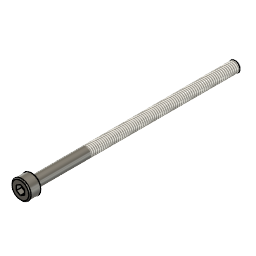
Equatorial Mount (Autodesk Fusion 360 archive; units mm, degrees)
design "Hexagon Socket Head Cap Screw ISO 4762 - M4 x 75 Steel 4.6 Plain"
description: Hexagon Socket Head Cap Screw ISO 4762 - M4 x 75
part number: ISO 4762 - M4 x 75 Steel 4.6 Plain
Autodesk Fusion 360 part; units mm, degrees
note: some values were not read from the file. Chosen so that the rebuilt part matches the saved one: how an offset face is resized. Set by a fixed rule: which face or edge a step refers to; which sketch regions a step uses.
sketch "Sketch1" plane through (0, 0, 0) normal (0, 1, 0) x (1, 0, 0)
  line L0 (-2, 0) -> (-2, 75)
  line L1 (-2, 75) -> (0, 75)
  line L2 (0, 75) -> (0, -4)
  line L3 (-2, 0) -> (-3.5, 0)
  line L4 (-3.5, 0) -> (-3.5, -4)
  line L5 (-3.5, -4) -> (0, -4)
  dimension "d9" = 4
  dimension "d106" = 4
  dimension "d107" = 75
  dimension "d116" = 7
  constraint perpendicular L0 L1
  constraint collinear origin L1.end L2.end
  constraint perpendicular L0 L3
  constraint coincident origin L3
  constraint vertical L2
  constraint coincident L2 L5.end
  constraint perpendicular L2 L5
  measures "d106" distance of L3 L5
  measures "d107" distance of origin L1
revolve "Revolve1" add sketch "Sketch1" angle 360 about axis through (0, 0, -75) along (0, 0, 1)
ref_plane "WorkPlane1" through (0, 0, 4) normal (0, 0, 1) x (1, 0, 0)
sketch "Sketch6" plane through (0, 0, 4) normal (0, 0, 1) x (1, 0, 0)
  line L0 (-1.5, 0.866) -> (-1.5, -0.866)
  line L1 (-1.5, -0.866) -> (0, -1.7321)
  line L2 (0, -1.7321) -> (1.5, -0.866)
  line L3 (1.5, -0.866) -> (1.5, 0.866)
  line L4 (1.5, 0.866) -> (0, 1.7321)
  line L5 (0, 1.7321) -> (-1.5, 0.866)
  dimension "d117" = 3
  constraint vertical L0
  measures "d117" distance of L0 L3
extrude "Extrude1" cut sketch "Sketch6" against normal blind 2
extrude "Extrude2" cut 1 faces at (0, -0.5774, 2) along direction (0, 0, -1) blind 2 draft -85
fillet "Fillet4" radius 0.4 1 edges at (-3.2631, 1.2657, 4)
thread "Thread3" "ISO Metric profile 4.0 M4x0.7 M4x0.7 6g" major diameter 3.908 minor diameter 3.111 pitch 0.7 angle 60 resizes the face on face at (-1.9901, 0.1991, -50)
sketch "Sketch7" plane through (0, 0, 0) normal (0, 1, 0) x (1, 0, 0)
  line L0 (-2.04, 75) -> (-2.04, 74.6)
  line L1 (-2.04, 74.6) -> (-1.64, 75)
  line L2 (0, 75) -> (0, -4)
  line L3 (-2.04, 75) -> (0, 75)
  dimension "d101" = 45
  dimension "d112" = 0.4
  dimension "d113" = 2.04
  constraint coincident L2.start L3.end
  constraint perpendicular L2 L3
  constraint coincident L1.end L3
  constraint perpendicular L0 L3
  measures "d101" angle of L0 L1
  measures "d112" distance of L0.end L3
  measures "d113" distance of L0 L2.start
revolve "Revolve3" cut sketch "Sketch7" angle 360 about axis through (0, 0, 1.75) along (0, 0, 1)
equation "d9 = adsk_nomdia"
equation "adsk_nomlen = 75.00 mm"
equation "adsk_headh = 4.00 mm"
equation "adsk_headdia = 7.00 mm"
equation "adsk_nomdia = 4.00 mm"
equation "adsk_philwidth = 3.00 mm"
equation "d31 = -adsk_phildepth"
equation "adsk_phildepth = 2.00 mm"
equation "d71 = adsk_headh"
equation "d76 = -adsk_phildepth"
equation "adsk_thrlen = 55.00 mm"
equation "d86 = adsk_nomdia * 0.1"
equation "adsk_startang = 45.00 deg"
equation "d101 = adsk_startang"
equation "adsk_pitch1 = 0.70 mm"
equation "adsk_startlen = 0.40 mm"
equation "d106 = adsk_headh"
equation "d107 = adsk_nomlen"
equation "d112 = adsk_startlen"
equation "d113 = adsk_nomdia * 0.51"
equation "d115 = min(adsk_thrlen; adsk_nomlen - 0.001 mm)"
equation "d116 = adsk_headdia"
equation "d117 = adsk_philwidth"

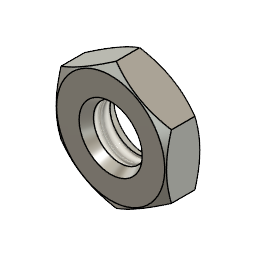
design "Hexagon Thin Nut ISO 4035 - M4 Steel 6 Plain"
description: Hexagon Thin Nut ISO 4035 - M4
part number: ISO 4035 - M4 Steel 6 Plain
Autodesk Fusion 360 part; units mm, degrees
sketch "Sketch1" plane through (0, 0, 0) normal (0, 1, 0) x (1, 0, 0)
  line L0 (0, 0) -> (0, -2.2)
  line L1 (-2, 0) -> (-3.43, 0)
  line L2 (-3.43, 0) -> (-4.0425, -0.3536)
  line L3 (-4.0425, -0.3536) -> (-4.0425, -1.8464)
  line L4 (-4.0425, -1.8464) -> (-3.43, -2.2)
  line L5 (-3.43, -2.2) -> (-2, -2.2)
  line L6 (-2, -2.2) -> (-2, 0)
  dimension "d121" = 4
  dimension "d122" = 30
  dimension "d123" = 30
  dimension "d128" = 8.085
  dimension "d172" = 6.86
  dimension "d179" = 2.2
  constraint vertical L0
  constraint coincident L0 L0.end
  constraint coincident origin L0
  constraint horizontal L1
  constraint coincident L0.start L1
  constraint coincident L0.start origin
  constraint coincident L0.end L5
  constraint vertical L1.end L4.end
  measures "d122" angle of L1 L2
  measures "d123" angle of L4 L5
  measures "d179" distance of L1 L5
revolve "Revolve1" add sketch "Sketch1" angle 360 about axis through (0, 0, 0) along (0, 0, 1)
sketch "Sketch8" plane through (0, 0, 2.2) normal (0, 0, 1) x (1, 0, 0)
  line L0 (-3.5, -2.0228) -> (-3.5, 2.0228)
  circle A0 centre (0, 0) radius 2
  circle A1 centre (0, 0) radius 4.0425
  dimension "d114" = 3.5
  constraint coincident L0.end A1
  constraint coincident L0.start A1
  constraint vertical L0
  measures "d114" distance of A0.centre L0
extrude "Extrude5" cut sketch "Sketch8" against normal blind 2.2 contours L0 A1 picked at (-3.5875, 0.4927)
pattern_circular "C-Pattern2" count 6 over 360 about axis through (0, 0, 1.75) along (0, 0, 1) of "Extrude5"
thread "Thread3" "ISO Metric profile 4.0 M4x0.7 M4x0.7 6H" major diameter 4.1095 minor diameter 3.332 pitch 0.7 angle 60 resizes the face on face at (-1.9975, 0.0997, 1.4667)
sketch "Sketch12" plane through (0, 0, 0) normal (0, 1, 0) x (1, 0, 0)
  line L0 (-2, 0) -> (0, 0)
  line L1 (-1.3649, -1.1) -> (-2, 0)
  line L2 (-2, -2.2) -> (0, -2.2)
  line L3 (-1.3649, -1.1) -> (-2, -2.2)
  line L4 (0, 0) -> (0, -2.2)
  dimension "d169" = 60
  dimension "d177" = 2
  dimension "d178" = 60
  constraint horizontal L0
  constraint coincident L1.start L3.start
  constraint vertical L0.start L2.start
  constraint coincident L2.end L4.end
  constraint coincident L0.end L4.start
  constraint perpendicular L2 L4
  measures "d169" angle of L2 L3
  measures "d177" distance of L0.start L4
  measures "d178" angle of L0 L1
revolve "Revolve3" cut sketch "Sketch12" angle 360 about axis through (0, 0, 1.75) along (0, 0, 1)
equation "adsk_nheig = 2.20 mm"
equation "adsk_maxdia = 8.085 mm"
equation "adsk_nomdia = 4.00 mm"
equation "d89 = -adsk_nheig"
equation "adsk_waflat = 7.00 mm"
equation "d114 = adsk_waflat / 2"
equation "adsk_chamang1 = 30.00 deg"
equation "adsk_chamang2 = 30.00 deg"
equation "d121 = adsk_nomdia"
equation "d122 = adsk_chamang1"
equation "d123 = adsk_chamang2"
equation "d128 = adsk_maxdia"
equation "d163 = adsk_nheig"
equation "adsk_beardia = 6.86 mm"
equation "d172 = adsk_beardia"
equation "d177 = adsk_nomdia * 0.5"
equation "d179 = adsk_nheig"

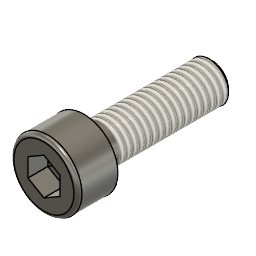
design "Hexagon Socket Head Cap Screw ISO 4762 - M5 x 16 Steel 4.6 Plain"
description: Hexagon Socket Head Cap Screw ISO 4762 - M5 x 16
part number: ISO 4762 - M5 x 16 Steel 4.6 Plain
Autodesk Fusion 360 part; units mm, degrees
sketch "Sketch1" plane through (0, 0, 0) normal (0, 1, 0) x (1, 0, 0)
  line L0 (-2.5, 0) -> (-2.5, 16)
  line L1 (-2.5, 16) -> (0, 16)
  line L2 (0, 16) -> (0, -5)
  line L3 (-2.5, 0) -> (-4.25, 0)
  line L4 (-4.25, 0) -> (-4.25, -5)
  line L5 (-4.25, -5) -> (0, -5)
  dimension "d9" = 5
  dimension "d106" = 5
  dimension "d107" = 16
  dimension "d116" = 8.5
  constraint perpendicular L0 L1
  constraint collinear origin L1.end L2.end
  constraint perpendicular L0 L3
  constraint coincident origin L3
  constraint vertical L2
  constraint coincident L2 L5.end
  constraint perpendicular L2 L5
  measures "d106" distance of L3 L5
  measures "d107" distance of origin L1
revolve "Revolve1" add sketch "Sketch1" angle 360 about axis through (0, 0, -16) along (0, 0, 1)
ref_plane "WorkPlane1" through (0, 0, 5) normal (0, 0, 1) x (1, 0, 0)
sketch "Sketch6" plane through (0, 0, 5) normal (0, 0, 1) x (1, 0, 0)
  line L0 (-2, 1.1547) -> (-2, -1.1547)
  line L1 (-2, -1.1547) -> (0, -2.3094)
  line L2 (0, -2.3094) -> (2, -1.1547)
  line L3 (2, -1.1547) -> (2, 1.1547)
  line L4 (2, 1.1547) -> (0, 2.3094)
  line L5 (0, 2.3094) -> (-2, 1.1547)
  dimension "d117" = 4
  constraint vertical L0
  measures "d117" distance of L0 L3
extrude "Extrude1" cut sketch "Sketch6" against normal blind 2.5
extrude "Extrude2" cut 1 faces at (0.6667, -0.3849, 2.5) along direction (0, 0, -1) blind 2.5 draft -85
fillet "Fillet4" radius 0.5 1 edges at (-3.9624, 1.5369, 5)
thread "Thread3" "ISO Metric profile 5.0 M5x0.8 M5x0.8 6g" major diameter 4.901 minor diameter 3.9895 pitch 0.8 angle 60 resizes the face on face at (-2.4876, 0.2489, -10.6667)
sketch "Sketch7" plane through (0, 0, 0) normal (0, 1, 0) x (1, 0, 0)
  line L0 (-2.55, 16) -> (-2.55, 15.5)
  line L1 (-2.55, 15.5) -> (-2.05, 16)
  line L2 (0, 16) -> (0, -5)
  line L3 (-2.55, 16) -> (0, 16)
  dimension "d101" = 45
  dimension "d112" = 0.5
  dimension "d113" = 2.55
  constraint coincident L2.start L3.end
  constraint perpendicular L2 L3
  constraint coincident L1.end L3
  constraint perpendicular L0 L3
  measures "d101" angle of L0 L1
  measures "d112" distance of L0.end L3
  measures "d113" distance of L0 L2.start
revolve "Revolve3" cut sketch "Sketch7" angle 360 about axis through (0, 0, 1.75) along (0, 0, 1)
equation "d9 = adsk_nomdia"
equation "adsk_nomlen = 16.00 mm"
equation "adsk_headh = 5.00 mm"
equation "adsk_headdia = 8.50 mm"
equation "adsk_nomdia = 5.00 mm"
equation "adsk_philwidth = 4.00 mm"
equation "d31 = -adsk_phildepth"
equation "adsk_phildepth = 2.50 mm"
equation "d71 = adsk_headh"
equation "d76 = -adsk_phildepth"
equation "adsk_thrlen = 14.00 mm"
equation "d86 = adsk_nomdia * 0.1"
equation "adsk_startang = 45.00 deg"
equation "d101 = adsk_startang"
equation "adsk_pitch1 = 0.80 mm"
equation "adsk_startlen = 0.50 mm"
equation "d106 = adsk_headh"
equation "d107 = adsk_nomlen"
equation "d112 = adsk_startlen"
equation "d113 = adsk_nomdia * 0.51"
equation "d115 = min(adsk_thrlen; adsk_nomlen - 0.001 mm)"
equation "d116 = adsk_headdia"
equation "d117 = adsk_philwidth"

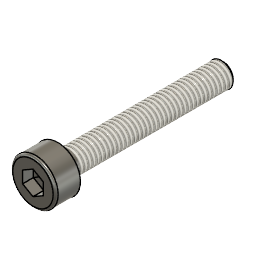
design "Hexagon Socket Head Cap Screw ISO 4762 - M3 x 20 Steel 4.6 Plain"
description: Hexagon Socket Head Cap Screw ISO 4762 - M3 x 20
part number: ISO 4762 - M3 x 20 Steel 4.6 Plain
Autodesk Fusion 360 part; units mm, degrees
sketch "Sketch1" plane through (0, 0, 0) normal (0, 1, 0) x (1, 0, 0)
  line L0 (-1.5, 0) -> (-1.5, 20)
  line L1 (-1.5, 20) -> (0, 20)
  line L2 (0, 20) -> (0, -3)
  line L3 (-1.5, 0) -> (-2.75, 0)
  line L4 (-2.75, 0) -> (-2.75, -3)
  line L5 (-2.75, -3) -> (0, -3)
  dimension "d9" = 3
  dimension "d106" = 3
  dimension "d107" = 20
  dimension "d116" = 5.5
  constraint perpendicular L0 L1
  constraint collinear origin L1.end L2.end
  constraint perpendicular L0 L3
  constraint coincident origin L3
  constraint vertical L2
  constraint coincident L2 L5.end
  constraint perpendicular L2 L5
  measures "d106" distance of L3 L5
  measures "d107" distance of origin L1
revolve "Revolve1" add sketch "Sketch1" angle 360 about axis through (0, 0, -20) along (0, 0, 1)
ref_plane "WorkPlane1" through (0, 0, 3) normal (0, 0, 1) x (1, 0, 0)
sketch "Sketch6" plane through (0, 0, 3) normal (0, 0, 1) x (1, 0, 0)
  line L0 (-1.25, 0.7217) -> (-1.25, -0.7217)
  line L1 (-1.25, -0.7217) -> (0, -1.4434)
  line L2 (0, -1.4434) -> (1.25, -0.7217)
  line L3 (1.25, -0.7217) -> (1.25, 0.7217)
  line L4 (1.25, 0.7217) -> (0, 1.4434)
  line L5 (0, 1.4434) -> (-1.25, 0.7217)
  dimension "d117" = 2.5
  constraint vertical L0
  measures "d117" distance of L0 L3
extrude "Extrude1" cut sketch "Sketch6" against normal blind 1.3
extrude "Extrude2" cut 1 faces at (-0.4167, 0.2406, 1.7) along direction (0, 0, -1) blind 1.3 draft -85
fillet "Fillet4" radius 0.3 1 edges at (-2.5639, 0.9944, 3)
thread "Thread3" "ISO Metric profile 3.0 M3x0.5 M3x0.5 6g" major diameter 2.927 minor diameter 2.3555 pitch 0.5 angle 60 resizes the face on face at (-1.4925, 0.1494, -13.3333)
sketch "Sketch7" plane through (0, 0, 0) normal (0, 1, 0) x (1, 0, 0)
  line L0 (-1.53, 20) -> (-1.53, 19.7)
  line L1 (-1.53, 19.7) -> (-1.23, 20)
  line L2 (0, 20) -> (0, -3)
  line L3 (-1.53, 20) -> (0, 20)
  dimension "d101" = 45
  dimension "d112" = 0.3
  dimension "d113" = 1.53
  constraint coincident L2.start L3.end
  constraint perpendicular L2 L3
  constraint coincident L1.end L3
  constraint perpendicular L0 L3
  measures "d101" angle of L0 L1
  measures "d112" distance of L0.end L3
  measures "d113" distance of L0 L2.start
revolve "Revolve3" cut sketch "Sketch7" angle 360 about axis through (0, 0, 1.75) along (0, 0, 1)
equation "d9 = adsk_nomdia"
equation "adsk_nomlen = 20.00 mm"
equation "adsk_headh = 3.00 mm"
equation "adsk_headdia = 5.50 mm"
equation "adsk_nomdia = 3.00 mm"
equation "adsk_philwidth = 2.50 mm"
equation "d31 = -adsk_phildepth"
equation "adsk_phildepth = 1.30 mm"
equation "d71 = adsk_headh"
equation "d76 = -adsk_phildepth"
equation "adsk_thrlen = 18.75 mm"
equation "d86 = adsk_nomdia * 0.1"
equation "adsk_startang = 45.00 deg"
equation "d101 = adsk_startang"
equation "adsk_pitch1 = 0.50 mm"
equation "adsk_startlen = 0.30 mm"
equation "d106 = adsk_headh"
equation "d107 = adsk_nomlen"
equation "d112 = adsk_startlen"
equation "d113 = adsk_nomdia * 0.51"
equation "d115 = min(adsk_thrlen; adsk_nomlen - 0.001 mm)"
equation "d116 = adsk_headdia"
equation "d117 = adsk_philwidth"

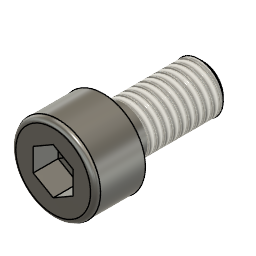
design "Hexagon Socket Head Cap Screw ISO 4762 - M5 x 10 Steel 4.6 Plain"
description: Hexagon Socket Head Cap Screw ISO 4762 - M5 x 10
part number: ISO 4762 - M5 x 10 Steel 4.6 Plain
Autodesk Fusion 360 part; units mm, degrees
sketch "Sketch1" plane through (0, 0, 0) normal (0, 1, 0) x (1, 0, 0)
  line L0 (-2.5, 0) -> (-2.5, 10)
  line L1 (-2.5, 10) -> (0, 10)
  line L2 (0, 10) -> (0, -5)
  line L3 (-2.5, 0) -> (-4.25, 0)
  line L4 (-4.25, 0) -> (-4.25, -5)
  line L5 (-4.25, -5) -> (0, -5)
  dimension "d9" = 5
  dimension "d106" = 5
  dimension "d107" = 10
  dimension "d116" = 8.5
  constraint perpendicular L0 L1
  constraint collinear origin L1.end L2.end
  constraint perpendicular L0 L3
  constraint coincident origin L3
  constraint vertical L2
  constraint coincident L2 L5.end
  constraint perpendicular L2 L5
  measures "d106" distance of L3 L5
  measures "d107" distance of origin L1
revolve "Revolve1" add sketch "Sketch1" angle 360 about axis through (0, 0, -10) along (0, 0, 1)
ref_plane "WorkPlane1" through (0, 0, 5) normal (0, 0, 1) x (1, 0, 0)
sketch "Sketch6" plane through (0, 0, 5) normal (0, 0, 1) x (1, 0, 0)
  line L0 (-2, 1.1547) -> (-2, -1.1547)
  line L1 (-2, -1.1547) -> (0, -2.3094)
  line L2 (0, -2.3094) -> (2, -1.1547)
  line L3 (2, -1.1547) -> (2, 1.1547)
  line L4 (2, 1.1547) -> (0, 2.3094)
  line L5 (0, 2.3094) -> (-2, 1.1547)
  dimension "d117" = 4
  constraint vertical L0
  measures "d117" distance of L0 L3
extrude "Extrude1" cut sketch "Sketch6" against normal blind 2.5
extrude "Extrude2" cut 1 faces at (0.6667, -0.3849, 2.5) along direction (0, 0, -1) blind 2.5 draft -85
fillet "Fillet4" radius 0.5 1 edges at (-3.9624, 1.5369, 5)
thread "Thread3" "ISO Metric profile 5.0 M5x0.8 M5x0.8 6g" major diameter 4.901 minor diameter 3.9895 pitch 0.8 angle 60 resizes the face on face at (-2.4876, 0.2489, -3.3333)
sketch "Sketch7" plane through (0, 0, 0) normal (0, 1, 0) x (1, 0, 0)
  line L0 (-2.55, 10) -> (-2.55, 9.5)
  line L1 (-2.55, 9.5) -> (-2.05, 10)
  line L2 (0, 10) -> (0, -5)
  line L3 (-2.55, 10) -> (0, 10)
  dimension "d101" = 45
  dimension "d112" = 0.5
  dimension "d113" = 2.55
  constraint coincident L2.start L3.end
  constraint perpendicular L2 L3
  constraint coincident L1.end L3
  constraint perpendicular L0 L3
  measures "d101" angle of L0 L1
  measures "d112" distance of L0.end L3
  measures "d113" distance of L0 L2.start
revolve "Revolve3" cut sketch "Sketch7" angle 360 about axis through (0, 0, 1.75) along (0, 0, 1)
equation "d9 = adsk_nomdia"
equation "adsk_nomlen = 10.00 mm"
equation "adsk_headh = 5.00 mm"
equation "adsk_headdia = 8.50 mm"
equation "adsk_nomdia = 5.00 mm"
equation "adsk_philwidth = 4.00 mm"
equation "d31 = -adsk_phildepth"
equation "adsk_phildepth = 2.50 mm"
equation "d71 = adsk_headh"
equation "d76 = -adsk_phildepth"
equation "adsk_thrlen = 8.00 mm"
equation "d86 = adsk_nomdia * 0.1"
equation "adsk_startang = 45.00 deg"
equation "d101 = adsk_startang"
equation "adsk_pitch1 = 0.80 mm"
equation "adsk_startlen = 0.50 mm"
equation "d106 = adsk_headh"
equation "d107 = adsk_nomlen"
equation "d112 = adsk_startlen"
equation "d113 = adsk_nomdia * 0.51"
equation "d115 = min(adsk_thrlen; adsk_nomlen - 0.001 mm)"
equation "d116 = adsk_headdia"
equation "d117 = adsk_philwidth"

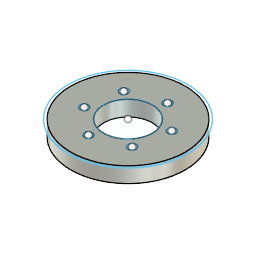
design "Bottom Output Plate"
Autodesk Fusion 360 part; units mm, degrees
sketch "sketch 334" plane through (0, 0, 6.35) normal (0, 0, -1) x (1, 0, 0)
  circle A0 centre (2.4311, 1.2127) radius 1.65
  circle A1 centre (10.7246, 23.999) radius 1.65
  circle A2 centre (-2.4311, 28.7873) radius 1.65
  circle A3 centre (-10.7246, 6.001) radius 1.65
  circle A4 centre (-13.1557, 19.7883) radius 1.65
  circle A5 centre (13.1557, 10.2117) radius 1.65
  circle A6 centre (0, 15) radius 10
  circle A7 centre (0, 15) radius 24.5
extrude "Extrude1" add sketch "sketch 334" along normal blind 6.35
move_face "OffsetFaces1" offset -1 1 faces at (24.3783, -12.5606, 2.1167)

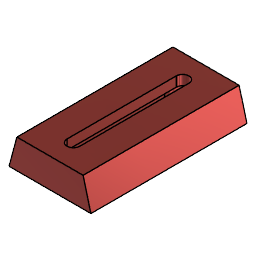
design "80mm Vixen Dovetail Bar"
Autodesk Fusion 360 part; units mm, degrees
sketch "Sketch1" plane through (0, 0, 0) normal (0, 1, 0) x (1, 0, 0)
  line L0 (0, 0) -> (42, 0)
  line L1 (21, 0) -> (21, -15)
  line L2 (0, 0) -> (4.0192, -15)
  line L3 (0, 0) -> (15.5291, 0) construction
  line L4 (4.0192, -15) -> (21, -15)
  line L5 (42, 0) -> (37.9808, -15)
  line L6 (21, -15) -> (37.9808, -15)
  dimension "d1" = 42
  dimension "d2" = 15
  dimension "d3" = 75
  dimension "d4" = 75
  constraint coincident L0.start L2.start
  constraint horizontal L0
  constraint midpoint L0 L1.start
  constraint perpendicular L0 L1
  constraint horizontal L3
  constraint perpendicular L1 L4
  constraint perpendicular L1 L6
  measures "d1" distance of L0.start L0.end
  measures "d2" distance of L1.start L1.end
  measures "d3" angle of L2 L3
  measures "d4" angle of L0 L5
extrude "Extrude1" add sketch "Sketch1" along normal blind 80
sketch "Sketch2" plane through (0, 0, 15) normal (0, 0, 1) x (-1, 0, 0)
  line L0 (-4.0192, 0) -> (-37.9808, 0)
  line L1 (-37.9808, 0) -> (-37.9808, -80)
  line L2 (-37.9808, -80) -> (-4.0192, -80)
  line L3 (-4.0192, -80) -> (-4.0192, 0)
  line L4 (-4.0192, -40) -> (-37.9808, -40)
  line L5 (-21, -40) -> (-21, -68)
  line L6 (-21, -40) -> (-21, -12)
  circle A0 centre (-21, -12) radius 3.25
  circle A1 centre (-21, -68) radius 3.25
  line L7 (-21, -68) -> (-17.75, -68)
  line L8 (-17.75, -68) -> (-17.75, -12)
  line L9 (-24.25, -12) -> (-24.25, -68)
  dimension "d7" = 28
  dimension "d8" = 28
  dimension "d9" = 6.5
  dimension "d10" = 6.5
  constraint midpoint L3 L4.start
  constraint midpoint L1 L4.end
  constraint midpoint L4 L5.start
  constraint perpendicular L4 L5
  constraint perpendicular L4 L6
  constraint coincident L6.end A0.centre
  constraint coincident L5.end A1.centre
  constraint coincident A1 L7.end
  constraint perpendicular L5 L7
  constraint coincident A0 L8.end
  constraint tangent A0 L8
  constraint coincident A0 L9.start
  constraint coincident A1 L9.end
  constraint tangent A1 L9
  constraint perpendicular L4 L9
  measures "d7" distance of L5.start L5.end
  measures "d8" distance of L5.start L6.end
  measures "d9" diameter of A0
  measures "d10" diameter of A1
extrude "Extrude2" cut sketch "Sketch2" against normal blind 15 contours L4 L5 A1 L8 | L4 L6 A0 L8 | L4 L6 A0 L9 | L4 L5 A1 L9 | L5 A1 L7 | L5 A1 L7 | A0
sketch "Sketch3" plane through (0, 0, 0) normal (0, 0, -1) x (1, 0, 0)
  arc A0 (17.75, -68) -> (24.25, -68) centre (21, -68) ccw
  line L0 (17.75, -68) -> (17.75, -12)
  arc A1 (24.25, -12) -> (17.75, -12) centre (21, -12) ccw
  line L1 (24.25, -12) -> (24.25, -68)
  line L2 (42, 0) -> (0, 0)
  line L3 (0, 0) -> (0, -80)
  line L4 (0, -80) -> (42, -80)
  line L5 (42, -80) -> (42, 0)
  line L6 (11.75, -68) -> (11.75, -12)
  arc A2 (30.25, -12) -> (11.75, -12) centre (21, -12) ccw
  line L7 (30.25, -12) -> (30.25, -68)
  arc A3 (11.75, -68) -> (30.25, -68) centre (21, -68) ccw
  dimension "d13" = 6
extrude "Extrude3" cut sketch "Sketch3" against normal blind 10 contours L6 A2 L7 A3

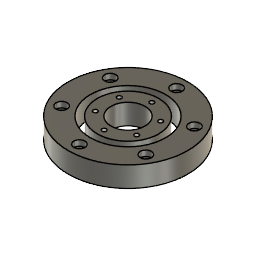
design "RU42UUCCO Slew Bearing"
Autodesk Fusion 360 part; units mm, degrees
sketch "Sketch1" plane through (0, 0, 0) normal (0, 0, 1) x (1, 0, 0)
  circle A0 centre (0, 0) radius 10
  circle A1 centre (0, 0) radius 35
  circle A2 centre (0, 0) radius 14
  circle A3 centre (0, 0) radius 18
  circle A4 centre (0, 0) radius 28.5
  line L0 (0, 0) -> (0, 35)
  circle A5 centre (0, 28.5) radius 3.25
  circle A6 centre (0, 14) radius 1.5
  circle A7 centre (-24.6817, 14.25) radius 3.25
  circle A8 centre (-24.6817, -14.25) radius 3.25
  circle A9 centre (0, -28.5) radius 3.25
  circle A10 centre (24.6817, -14.25) radius 3.25
  circle A11 centre (24.6817, 14.25) radius 3.25
  circle A12 centre (-12.1244, 7) radius 1.5
  circle A13 centre (-12.1244, -7) radius 1.5
  circle A14 centre (0, -14) radius 1.5
  circle A15 centre (12.1244, -7) radius 1.5
  circle A16 centre (12.1244, 7) radius 1.5
  line L1 (0, 28.5) -> (0, 22)
  circle A17 centre (0, 0) radius 22
  circle A18 centre (0, 28.5) radius 1.65
  circle A19 centre (-24.6817, 14.25) radius 1.65
  circle A20 centre (-24.6817, -14.25) radius 1.65
  circle A21 centre (0, -28.5) radius 1.65
  circle A22 centre (24.6817, -14.25) radius 1.65
  circle A23 centre (24.6817, 14.25) radius 1.65
  dimension "d1" = 20
  dimension "d2" = 70
  dimension "d3" = 28
  dimension "d4" = 36
  dimension "d5" = 57
  dimension "d6" = 6.5
  dimension "d7" = 3
  dimension "d9" = 360
  dimension "d11" = 360
  dimension "d12" = 6.5
  dimension "d17" = 3.3
  dimension "d19" = 360
  constraint coincident A0.centre A1.centre
  constraint concentric A0 A3
  constraint concentric A2 A4
  constraint coincident A1 L0.end
  constraint vertical L0
  constraint coincident A4 A5.centre
  constraint coincident L0 A5.centre
  constraint coincident L0 A6.centre
  constraint coincident A5.centre L1.start
  constraint parallel L0 L1
  constraint concentric A3 A17
  constraint coincident L1.end A17
  constraint concentric A5 A18
  measures "d1" diameter of A0
  measures "d2" diameter of A1
  measures "d3" diameter of A2
  measures "d4" diameter of A3
  measures "d5" diameter of A4
  measures "d6" diameter of A5
  measures "d7" diameter of A6
  measures "d12" distance of A5.centre L1.end
  measures "d17" diameter of A18
extrude "Extrude1" add sketch "Sketch1" along normal blind 12 contours A2 A6 A12 A13 A14 A15 A16 | A3 makes body 1
extrude "Extrude2" add sketch "Sketch1" along normal blind 12 separate body contours A1 | A4 A5 A7 A8 A9 A10 A11 makes body 2
extrude "Extrude3" add sketch "Sketch1" along normal blind 8.7 contours A4 A11 A23 | A4 A11 A23 | A4 A10 A22 | A4 A10 A22 | A4 L0 A5 L1 A18 | A4 L0 A5 A18 | A4 A9 A21 | A4 A9 A21 | A4 L0 A5 L1 A18 | A4 L0 A5 A18 | A4 A8 A20 | A4 A8 A20 | A4 A7 A19 | A4 A7 A19 bodies 2
thread "Thread1" "ISO Metric profile 3.0 M3x0.5 M3x0.5 6H" major diameter 3.086 minor diameter 2.529 pitch 0.5 angle 60 resizes the face on face at (11.3668, -8.2946, 4) on face at (-11.3687, 8.2957, 4) on face at (1.02, -15.0998, 4) on face at (1.4996, 13.9643, 8) on face at (12.8643, 5.6952, 4) on face at (-11.4334, -8.3314, 8) on bodies 1
equation "d20 = 12.00 mm - 3.3 mm"

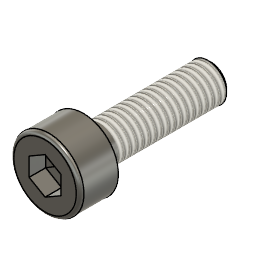
design "Hexagon Socket Head Cap Screw ISO 4762 - M3 x 10 Steel 4.6 Plain"
description: Hexagon Socket Head Cap Screw ISO 4762 - M3 x 10
part number: ISO 4762 - M3 x 10 Steel 4.6 Plain
Autodesk Fusion 360 part; units mm, degrees
sketch "Sketch1" plane through (0, 0, 0) normal (0, 1, 0) x (1, 0, 0)
  line L0 (-1.5, 0) -> (-1.5, 10)
  line L1 (-1.5, 10) -> (0, 10)
  line L2 (0, 10) -> (0, -3)
  line L3 (-1.5, 0) -> (-2.75, 0)
  line L4 (-2.75, 0) -> (-2.75, -3)
  line L5 (-2.75, -3) -> (0, -3)
  dimension "d9" = 3
  dimension "d106" = 3
  dimension "d107" = 10
  dimension "d116" = 5.5
  constraint perpendicular L0 L1
  constraint collinear origin L1.end L2.end
  constraint perpendicular L0 L3
  constraint coincident origin L3
  constraint vertical L2
  constraint coincident L2 L5.end
  constraint perpendicular L2 L5
  measures "d106" distance of L3 L5
  measures "d107" distance of origin L1
revolve "Revolve1" add sketch "Sketch1" angle 360 about axis through (0, 0, -10) along (0, 0, 1)
ref_plane "WorkPlane1" through (0, 0, 3) normal (0, 0, 1) x (1, 0, 0)
sketch "Sketch6" plane through (0, 0, 3) normal (0, 0, 1) x (1, 0, 0)
  line L0 (-1.25, 0.7217) -> (-1.25, -0.7217)
  line L1 (-1.25, -0.7217) -> (0, -1.4434)
  line L2 (0, -1.4434) -> (1.25, -0.7217)
  line L3 (1.25, -0.7217) -> (1.25, 0.7217)
  line L4 (1.25, 0.7217) -> (0, 1.4434)
  line L5 (0, 1.4434) -> (-1.25, 0.7217)
  dimension "d117" = 2.5
  constraint vertical L0
  measures "d117" distance of L0 L3
extrude "Extrude1" cut sketch "Sketch6" against normal blind 1.3
extrude "Extrude2" cut 1 faces at (-0.4167, 0.2406, 1.7) along direction (0, 0, -1) blind 1.3 draft -85
fillet "Fillet4" radius 0.3 1 edges at (-2.5639, 0.9944, 3)
thread "Thread3" "ISO Metric profile 3.0 M3x0.5 M3x0.5 6g" major diameter 2.927 minor diameter 2.3555 pitch 0.5 angle 60 resizes the face on face at (-1.4925, 0.1494, -6.6667)
sketch "Sketch7" plane through (0, 0, 0) normal (0, 1, 0) x (1, 0, 0)
  line L0 (-1.53, 10) -> (-1.53, 9.7)
  line L1 (-1.53, 9.7) -> (-1.23, 10)
  line L2 (0, 10) -> (0, -3)
  line L3 (-1.53, 10) -> (0, 10)
  dimension "d101" = 45
  dimension "d112" = 0.3
  dimension "d113" = 1.53
  constraint coincident L2.start L3.end
  constraint perpendicular L2 L3
  constraint coincident L1.end L3
  constraint perpendicular L0 L3
  measures "d101" angle of L0 L1
  measures "d112" distance of L0.end L3
  measures "d113" distance of L0 L2.start
revolve "Revolve3" cut sketch "Sketch7" angle 360 about axis through (0, 0, 1.75) along (0, 0, 1)
equation "d9 = adsk_nomdia"
equation "adsk_nomlen = 10.00 mm"
equation "adsk_headh = 3.00 mm"
equation "adsk_headdia = 5.50 mm"
equation "adsk_nomdia = 3.00 mm"
equation "adsk_philwidth = 2.50 mm"
equation "d31 = -adsk_phildepth"
equation "adsk_phildepth = 1.30 mm"
equation "d71 = adsk_headh"
equation "d76 = -adsk_phildepth"
equation "adsk_thrlen = 8.75 mm"
equation "d86 = adsk_nomdia * 0.1"
equation "adsk_startang = 45.00 deg"
equation "d101 = adsk_startang"
equation "adsk_pitch1 = 0.50 mm"
equation "adsk_startlen = 0.30 mm"
equation "d106 = adsk_headh"
equation "d107 = adsk_nomlen"
equation "d112 = adsk_startlen"
equation "d113 = adsk_nomdia * 0.51"
equation "d115 = min(adsk_thrlen; adsk_nomlen - 0.001 mm)"
equation "d116 = adsk_headdia"
equation "d117 = adsk_philwidth"

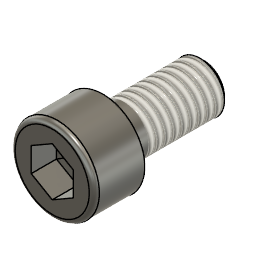
design "Hexagon Socket Head Cap Screw ISO 4762 - M6 x 12 Steel 4.6 Plain"
description: Hexagon Socket Head Cap Screw ISO 4762 - M6 x 12
part number: ISO 4762 - M6 x 12 Steel 4.6 Plain
Autodesk Fusion 360 part; units mm, degrees
sketch "Sketch1" plane through (0, 0, 0) normal (0, 1, 0) x (1, 0, 0)
  line L0 (-3, 0) -> (-3, 12)
  line L1 (-3, 12) -> (0, 12)
  line L2 (0, 12) -> (0, -6)
  line L3 (-3, 0) -> (-5, 0)
  line L4 (-5, 0) -> (-5, -6)
  line L5 (-5, -6) -> (0, -6)
  dimension "d9" = 6
  dimension "d106" = 6
  dimension "d107" = 12
  dimension "d116" = 10
  constraint perpendicular L0 L1
  constraint collinear origin L1.end L2.end
  constraint perpendicular L0 L3
  constraint coincident origin L3
  constraint vertical L2
  constraint coincident L2 L5.end
  constraint perpendicular L2 L5
  measures "d106" distance of L3 L5
  measures "d107" distance of origin L1
revolve "Revolve1" add sketch "Sketch1" angle 360 about axis through (0, 0, -12) along (0, 0, 1)
ref_plane "WorkPlane1" through (0, 0, 6) normal (0, 0, 1) x (1, 0, 0)
sketch "Sketch6" plane through (0, 0, 6) normal (0, 0, 1) x (1, 0, 0)
  line L0 (-2.5, 1.4434) -> (-2.5, -1.4434)
  line L1 (-2.5, -1.4434) -> (0, -2.8868)
  line L2 (0, -2.8868) -> (2.5, -1.4434)
  line L3 (2.5, -1.4434) -> (2.5, 1.4434)
  line L4 (2.5, 1.4434) -> (0, 2.8868)
  line L5 (0, 2.8868) -> (-2.5, 1.4434)
  dimension "d117" = 5
  constraint vertical L0
  measures "d117" distance of L0 L3
extrude "Extrude1" cut sketch "Sketch6" against normal blind 3
extrude "Extrude2" cut 1 faces at (0, -0.9623, 3) along direction (0, 0, -1) blind 3 draft -85
fillet "Fillet4" radius 0.6 1 edges at (-4.6616, 1.8081, 6)
thread "Thread3" "ISO Metric profile 6.0 M6x1 M6x1 6g" major diameter 5.884 minor diameter 4.7435 pitch 1 angle 60 resizes the face on face at (-2.9851, 0.2987, -8)
sketch "Sketch7" plane through (0, 0, 0) normal (0, 1, 0) x (1, 0, 0)
  line L0 (-3.06, 12) -> (-3.06, 11.4)
  line L1 (-3.06, 11.4) -> (-2.46, 12)
  line L2 (0, 12) -> (0, -6)
  line L3 (-3.06, 12) -> (0, 12)
  dimension "d101" = 45
  dimension "d112" = 0.6
  dimension "d113" = 3.06
  constraint coincident L2.start L3.end
  constraint perpendicular L2 L3
  constraint coincident L1.end L3
  constraint perpendicular L0 L3
  measures "d101" angle of L0 L1
  measures "d112" distance of L0.end L3
  measures "d113" distance of L0 L2.start
revolve "Revolve3" cut sketch "Sketch7" angle 360 about axis through (0, 0, 1.75) along (0, 0, 1)
equation "d9 = adsk_nomdia"
equation "adsk_nomlen = 12.00 mm"
equation "adsk_headh = 6.00 mm"
equation "adsk_headdia = 10.00 mm"
equation "adsk_nomdia = 6.00 mm"
equation "adsk_philwidth = 5.00 mm"
equation "d31 = -adsk_phildepth"
equation "adsk_phildepth = 3.00 mm"
equation "d71 = adsk_headh"
equation "d76 = -adsk_phildepth"
equation "adsk_thrlen = 9.50 mm"
equation "d86 = adsk_nomdia * 0.1"
equation "adsk_startang = 45.00 deg"
equation "d101 = adsk_startang"
equation "adsk_pitch1 = 1.00 mm"
equation "adsk_startlen = 0.60 mm"
equation "d106 = adsk_headh"
equation "d107 = adsk_nomlen"
equation "d112 = adsk_startlen"
equation "d113 = adsk_nomdia * 0.51"
equation "d115 = min(adsk_thrlen; adsk_nomlen - 0.001 mm)"
equation "d116 = adsk_headdia"
equation "d117 = adsk_philwidth"
